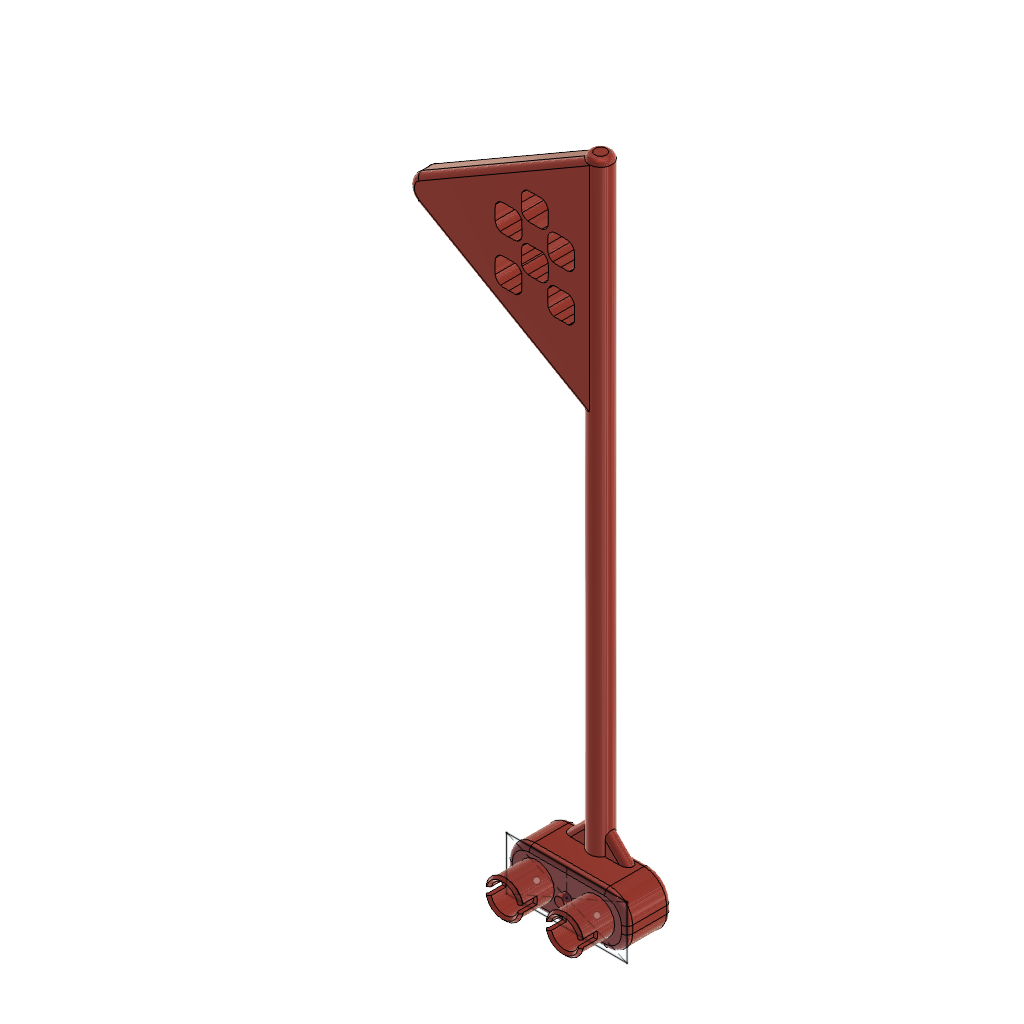
roversa_flag (Autodesk Fusion 360 design; units mm, degrees)
part number: 2026-09-13-09-05-21-145
Autodesk Fusion 360 part; units mm, degrees
sketch "Sketch1" plane through (0, 0, 0) normal (0, 1, 0) x (1, 0, 0)
  line L0 (8, -3.5) -> (-8, -3.5)
  line L1 (-8, -3.5) -> (-8, 3.5)
  line L2 (-8, 3.5) -> (8, 3.5)
  line L3 (8, 3.5) -> (8, -3.5)
  line L4 (8, -3.5) -> (-8, 3.5) construction
  line L5 (-8, -3.5) -> (8, 3.5) construction
  line L6 (0, -3.5) -> (0, 3.5) construction
  point P0 (-4, 0)
  point P1 (4, 0)
  dimension "d9" = 16
  dimension "d10" = 7
  dimension "d11" = 8
  constraint horizontal L0
  constraint perpendicular L0 L1
  constraint parallel L0 L2
  constraint parallel L1 L3
  constraint coincident L4 origin
  constraint coincident L5 origin
  constraint midpoint L0 L6.start
  constraint midpoint L2 L6.end
  constraint symmetric P0 P1 L6
  measures "d9" distance of L1.end L2.end
  measures "d10" distance of L0.end L1.end
  measures "d11" distance of P0 P1
extrude "Extrude1" add sketch "Sketch1" along normal blind 6
sketch "Sketch2" plane through (0, 0, 0) normal (0, 1, 0) x (1, 0, 0)
  circle A0 centre (-4, 0) radius 2.35
  circle A1 centre (-4, 0) radius 1.85
  dimension "d15" = 4.7
  dimension "d16" = 3.7
  constraint concentric A0 A1
  measures "d15" diameter of A0
  measures "d16" diameter of A1
extrude "Extrude2" add sketch "Sketch2" against normal blind 4.25
sketch "Sketch3" plane through (0, 0, 0) normal (0, 1, 0) x (1, 0, 0)
  circle A0 centre (4, 0) radius 2.35
  circle A1 centre (4, 0) radius 1.85
  dimension "d20" = 4.7
  dimension "d21" = 3.7
  constraint concentric A0 A1
  measures "d20" diameter of A0
  measures "d21" diameter of A1
extrude "Extrude3" add sketch "Sketch3" against normal blind 4.25
sketch "Sketch4" plane through (0, -4.25, 0) normal (0, -1, 0) x (1, 0, 0)
  circle A0 centre (-4, 0) radius 1.85
  circle A1 centre (-4, 0) radius 2.35
  circle A2 centre (-4, 0) radius 2.5
  dimension "d25" = 0.15
extrude "Extrude4" add sketch "Sketch4" along normal blind 1 draft -45 contours A1 | A2
sketch "Sketch5" plane through (0, -4.25, 0) normal (0, -1, 0) x (1, 0, 0)
  circle A0 centre (4, 0) radius 1.85
  circle A1 centre (4, 0) radius 2.35
  circle A2 centre (4, 0) radius 2.5
  dimension "d28" = 0.15
extrude "Extrude5" add sketch "Sketch5" along normal blind 1 draft -45 contours A1 | A2
ref_plane "WorkPlane1" through (-4, -4.575, 2.175) normal (0, 1, 0) x (-1, 0, 0)
sketch "Sketch6" plane through (0, -4.575, 0) normal (0, 1, 0) x (1, 0, 0)
  line L0 (-7.4125, -0.5) -> (-0.3625, -0.5)
  line L1 (-0.3625, -0.5) -> (-0.3625, 0.5)
  line L2 (-0.3625, 0.5) -> (-7.4125, 0.5)
  line L3 (-7.4125, 0.5) -> (-7.4125, -0.5)
  line L4 (-7.4125, -0.5) -> (-0.3625, 0.5) construction
  line L5 (-0.3625, -0.5) -> (-7.4125, 0.5) construction
  point P0 (-3.8875, 0)
  dimension "d32" = 1
  dimension "d33" = 7.05
  constraint horizontal L0
  constraint perpendicular L0 L1
  constraint parallel L0 L2
  constraint parallel L1 L3
  constraint coincident L4 P0
  constraint coincident L5 P0
  measures "d32" distance of L0.end L1.end
  measures "d33" distance of L0.start L0.end
extrude "Extrude6" cut sketch "Sketch6" along normal blind 2.3
sketch "Sketch7" plane through (0, -4.575, 0) normal (0, 1, 0) x (1, 0, 0)
  line L0 (0.5875, -0.5) -> (7.6375, -0.5)
  line L1 (7.6375, -0.5) -> (7.6375, 0.5)
  line L2 (7.6375, 0.5) -> (0.5875, 0.5)
  line L3 (0.5875, 0.5) -> (0.5875, -0.5)
  line L4 (0.5875, -0.5) -> (7.6375, 0.5) construction
  line L5 (7.6375, -0.5) -> (0.5875, 0.5) construction
  point P0 (4.1125, 0)
  dimension "d36" = 7.05
  dimension "d37" = 1
  constraint horizontal L0
  constraint perpendicular L0 L1
  constraint parallel L0 L2
  constraint parallel L1 L3
  constraint coincident L4 P0
  constraint coincident L5 P0
  measures "d36" distance of L0.start L0.end
  measures "d37" distance of L0.start L2.end
extrude "Extrude7" cut sketch "Sketch7" along normal blind 2.3
fillet "Fillet1" radius 3 4 edges at (8, 3, 3.5) (-8, 3, 3.5) (-8, 3, -3.5) (8, 3, -3.5)
sketch "Sketch8" plane through (0, 0, 3.5) normal (0, 0, 1) x (-1, 0, 0)
  line L0 (5, -6) -> (5, 0)
  line L1 (5, 0) -> (-5, 0)
  line L2 (-5, 0) -> (-5, -6)
  line L3 (-5, -6) -> (5, -6)
  circle A0 centre (0, -4.5) radius 1.5
  dimension "d45" = 3
  constraint tangent L3 A0
  measures "d45" diameter of A0
extrude "Extrude8" add sketch "Sketch8" along normal blind 80 contours A0
sketch "Sketch9" plane through (0, 6, 0) normal (0, 1, 0) x (-1, 0, 0)
  arc A0 (-8, -0.5) -> (-5, -3.5) centre (-5, -0.5) ccw
  line L0 (-5, -3.5) -> (5, -3.5)
  arc A1 (5, -3.5) -> (8, -0.5) centre (5, -0.5) ccw
  line L1 (8, -0.5) -> (8, 0.5)
  arc A2 (8, 0.5) -> (5, 3.5) centre (5, 0.5) ccw
  line L2 (5, 3.5) -> (0, 3.5)
  line L3 (0, 3.5) -> (-5, 3.5)
  arc A3 (-5, 3.5) -> (-8, 0.5) centre (-5, 0.5) ccw
  line L4 (-8, 0.5) -> (-8, -0.5)
  line L5 (0, 83.5) -> (25.9808, 68.5)
  line L6 (0, 83.5) -> (8.2765, 83.5) construction
  line L7 (25.9808, 68.5) -> (0, 53.5)
  line L8 (25.9808, 68.5) -> (15.4835, 68.5) construction
  line L9 (0, 53.5) -> (0, 83.5)
  line L10 (1.5, 83.5) -> (-1.5, 83.5)
  line L11 (-1.5, 3.5) -> (-1.5, 83.5)
  line L12 (-5, 3.5) -> (-1.5, 3.5)
  arc A4 (-5, 3.5) -> (-8, 0.5) centre (-5, 0.5) ccw
  line L13 (-8, -0.5) -> (-8, 0.5)
  arc A5 (-8, -0.5) -> (-5, -3.5) centre (-5, -0.5) ccw
  line L14 (5, -3.5) -> (-5, -3.5)
  arc A6 (5, -3.5) -> (8, -0.5) centre (5, -0.5) ccw
  line L15 (8, 0.5) -> (8, -0.5)
  arc A7 (8, 0.5) -> (5, 3.5) centre (5, 0.5) ccw
  line L16 (1.5, 3.5) -> (5, 3.5)
  line L17 (1.5, 3.5) -> (1.5, 83.5)
  point P0 (0, 83.5)
  dimension "d50" = 30
  dimension "d51" = 150
  dimension "d55" = 30
  constraint horizontal L6
  constraint horizontal L8
  constraint perpendicular L6 L9
  constraint midpoint L10 P0
  constraint coincident P0 L5.start
  measures "d50" angle of L5 L6
  measures "d51" angle of L7 L8
  measures "d55" distance of P0 L7.end
extrude "Extrude9" add sketch "Sketch9" against normal blind 3 contours L5 L7 L9 L17 | L5 L7 L17
fillet "Fillet3" radius 0.75 17 edges at (7.1213, 6, 2.6213) (8, 6, 0) (7.1213, 6, -2.6213) (0, 6, -3.5) (-7.1213, 6, -2.6213) (-8, 6, 0) (-7.1213, 6, 2.6213) (-2.5, 6, 3.5) (2.5, 6, 3.5) (-7.1213, 0, 2.6213) (-8, 0, 0) (-7.1213, 0, -2.6213) (0, 0, -3.5) (7.1213, 0, -2.6213) (8, 0, 0) (7.1213, 0, 2.6213) (0, 0, 3.5)
chamfer "Chamfer1" distance 0.15 angle 45 1 edges at (-4, -4.25, 2.35)
chamfer "Chamfer2" distance 0.15 angle 45 1 edges at (-4, -4.25, -2.35)
chamfer "Chamfer3" distance 0.15 angle 45 1 edges at (4, -4.25, -2.35)
chamfer "Chamfer4" distance 0.15 angle 45 1 edges at (4, -4.25, 2.35)
sketch "Sketch10" plane through (0, 0, 0) normal (0, 1, 0) x (1, 0, 0)
  circle A0 centre (0, 0) radius 0.65
  dimension "d66" = 1.3
  constraint coincident A0.centre origin
  measures "d66" diameter of A0
extrude "Extrude10" add sketch "Sketch10" against normal blind 1
ref_plane "WorkPlane2" through (0, 5.25, 0.375) normal (0, 1, 0) x (0, 0, 1)
sketch "Sketch11" plane through (0, 5.25, 0) normal (0, 1, 0) x (1, 0, 0)
  line L0 (-4.3507, -3.4546) -> (-1.3507, -3.4546)
  line L1 (-1.3507, -3.4546) -> (-1.3507, -6.4546)
  line L2 (-1.3507, -6.4546) -> (-4.3507, -3.4546)
  line L3 (-5, -3.5) -> (4.5424, -3.229) construction
  line L4 (4.5424, -3.229) -> (5, -3.5) construction
  line L5 (0, -3.5) -> (0, -6.024) construction
  line L6 (1.3507, -3.4546) -> (1.3507, -6.4546)
  line L7 (1.3507, -6.4546) -> (4.3507, -3.4546)
  line L8 (4.3507, -3.4546) -> (1.3507, -3.4546)
  dimension "d71" = 45
  dimension "d72" = 3
  constraint horizontal L0
  constraint perpendicular L0 L1
  constraint vertical L5
  constraint symmetric L0.start L5 L7.end
  constraint symmetric L0.end L5 L6.start
  constraint symmetric L1.end L5 L6.end
  measures "d71" angle of L1 L2
  measures "d72" distance of L0.start L0.end
extrude "Extrude11" add sketch "Sketch11" against normal blind 1.5
fillet "Fillet4" radius 0.75 4 edges at (2.8281, 5.25, 4.9773) (-2.8281, 5.25, 4.9773) (-2.8281, 3.75, 4.9773) (2.8281, 3.75, 4.9773)
fillet "Fillet5" radius 0.75 4 edges at (-12.9904, 6, 61) (-12.9904, 3, 61) (-12.9904, 6, 76) (-12.9904, 3, 76)
fillet "Fillet6" radius 0.75 1 edges at (1.3985, 5.0424, 83.5)
fillet "Fillet7" radius 2 3 edges at (-25.5414, 5.7803, 68.5) (-25.9808, 4.5, 68.5) (-25.5414, 3.2197, 68.5)
sketch "roversa-icon" plane through (0, 3, 0) normal (0, -1, 0) x (0, 0, -1)
  line L0 (-77.6583, 1.3985) -> (-77.6583, -15.6015)
  line L1 (-60.6583, -15.6015) -> (-60.6583, 1.3985)
  line L2 (-77.6583, -15.6015) -> (-60.6583, -15.6015)
  line L3 (-60.6583, 1.3985) -> (-77.6583, 1.3985)
  spline S0 degree 3 poles (-63.0001, -11.796) (-63.1468, -12.1963) (-63.447, -12.4351) (-63.89, -12.5038) knots 0 0 0 0 1 1 1 1
  spline S1 degree 3 poles (-63.89, -12.5038) (-64.2458, -12.559) (-65.6097, -12.527) (-65.7914, -12.4591) knots 0 0 0 0 1 1 1 1
  spline S2 degree 3 poles (-65.7914, -12.4591) (-66.1335, -12.3314) (-66.4173, -12.0056) (-66.4895, -11.6575) knots 0 0 0 0 1 1 1 1
  spline S3 degree 3 poles (-66.4895, -11.6575) (-66.5121, -11.5487) (-66.5212, -11.176) (-66.5147, -10.6238) knots 0 0 0 0 1 1 1 1
  spline S4 degree 3 poles (-66.5147, -10.6238) (-66.505, -9.8046) (-66.5008, -9.7523) (-66.4326, -9.6044) knots 0 0 0 0 1 1 1 1
  spline S5 degree 3 poles (-66.4326, -9.6044) (-66.3229, -9.3666) (-66.1659, -9.1969) (-65.9446, -9.0769) knots 0 0 0 0 1 1 1 1
  line L4 (-65.9446, -9.0769) -> (-65.7439, -8.9681)
  line L5 (-65.7439, -8.9681) -> (-64.7298, -8.9681)
  spline S6 degree 3 poles (-64.7298, -8.9681) (-63.7415, -8.9681) (-63.712, -8.9699) (-63.5707, -9.0395) knots 0 0 0 0 1 1 1 1
  spline S7 degree 3 poles (-63.5707, -9.0395) (-63.3477, -9.1494) (-63.1831, -9.3081) (-63.0638, -9.5282) knots 0 0 0 0 1 1 1 1
  line L6 (-63.0638, -9.5282) -> (-62.9551, -9.7287)
  line L7 (-62.9551, -9.7287) -> (-62.9472, -10.6794)
  spline S8 degree 3 poles (-62.9472, -10.6794) (-62.94, -11.5494) (-62.9445, -11.6442) (-63.0001, -11.796) knots 0 0 0 0 1 1 1 1
  spline S9 degree 3 poles (-62.9681, -4.7234) (-63.04, -5.013) (-63.2796, -5.2988) (-63.5707, -5.4423) knots 0 0 0 0 1 1 1 1
  spline S10 degree 3 poles (-63.5707, -5.4423) (-63.712, -5.5119) (-63.7415, -5.5137) (-64.7298, -5.5137) knots 0 0 0 0 1 1 1 1
  line L8 (-64.7298, -5.5137) -> (-65.7439, -5.5137)
  line L9 (-65.7439, -5.5137) -> (-65.9114, -5.4255)
  spline S11 degree 3 poles (-65.9114, -5.4255) (-66.1348, -5.3078) (-66.3183, -5.1185) (-66.4206, -4.9004) knots 0 0 0 0 1 1 1 1
  line L10 (-66.4206, -4.9004) -> (-66.5045, -4.7214)
  line L11 (-66.5045, -4.7214) -> (-66.5045, -3.7542)
  line L12 (-66.5045, -3.7542) -> (-66.5045, -2.7869)
  line L13 (-66.5045, -2.7869) -> (-66.4003, -2.5753)
  spline S12 degree 3 poles (-66.4003, -2.5753) (-66.2758, -2.3225) (-66.0808, -2.1389) (-65.8278, -2.0366) knots 0 0 0 0 1 1 1 1
  spline S13 degree 3 poles (-65.8278, -2.0366) (-65.6555, -1.967) (-65.6141, -1.9643) (-64.7139, -1.9643) knots 0 0 0 0 1 1 1 1
  line L14 (-64.7139, -1.9643) -> (-63.779, -1.9643)
  line L15 (-63.779, -1.9643) -> (-63.5992, -2.0486)
  spline S14 degree 3 poles (-63.5992, -2.0486) (-63.3587, -2.1613) (-63.1499, -2.3599) (-63.0429, -2.5777) knots 0 0 0 0 1 1 1 1
  line L16 (-63.0429, -2.5777) -> (-62.9551, -2.7566)
  line L17 (-62.9551, -2.7566) -> (-62.9495, -3.6915)
  spline S15 degree 3 poles (-62.9495, -3.6915) (-62.9465, -4.2057) (-62.9548, -4.67) (-62.9681, -4.7234) knots 0 0 0 0 1 1 1 1
  spline S16 degree 3 poles (-66.0446, -8.147) (-66.1116, -8.4683) (-66.3324, -8.7578) (-66.6313, -8.9159) knots 0 0 0 0 1 1 1 1
  line L18 (-66.6313, -8.9159) -> (-66.7897, -8.9998)
  line L19 (-66.7897, -8.9998) -> (-67.7586, -9.0093)
  spline S17 degree 3 poles (-67.7586, -9.0093) (-68.679, -9.0184) (-68.7364, -9.0156) (-68.9059, -8.9522) knots 0 0 0 0 1 1 1 1
  spline S18 degree 3 poles (-68.9059, -8.9522) (-69.1279, -8.8691) (-69.3617, -8.6624) (-69.4847, -8.4404) knots 0 0 0 0 1 1 1 1
  line L20 (-69.4847, -8.4404) -> (-69.5786, -8.2709)
  line L21 (-69.5786, -8.2709) -> (-69.5786, -7.2409)
  line L22 (-69.5786, -7.2409) -> (-69.5786, -6.2109)
  line L23 (-69.5786, -6.2109) -> (-69.4857, -6.0433)
  spline S19 degree 3 poles (-69.4857, -6.0433) (-69.3794, -5.8515) (-69.1831, -5.6586) (-68.998, -5.5642) knots 0 0 0 0 1 1 1 1
  spline S20 degree 3 poles (-68.998, -5.5642) (-68.7852, -5.4556) (-68.4723, -5.4271) (-67.6485, -5.4412) knots 0 0 0 0 1 1 1 1
  spline S21 degree 3 poles (-67.6485, -5.4412) (-66.9969, -5.4524) (-66.8639, -5.463) (-66.7422, -5.5131) knots 0 0 0 0 1 1 1 1
  spline S22 degree 3 poles (-66.7422, -5.5131) (-66.4321, -5.641) (-66.2217, -5.8512) (-66.0911, -6.1634) knots 0 0 0 0 1 1 1 1
  spline S23 degree 3 poles (-66.0911, -6.1634) (-66.0384, -6.2894) (-66.0307, -6.4054) (-66.0245, -7.1617) knots 0 0 0 0 1 1 1 1
  spline S24 degree 3 poles (-66.0245, -7.1617) (-66.0207, -7.6323) (-66.0298, -8.0757) (-66.0446, -8.147) knots 0 0 0 0 1 1 1 1
  spline S25 degree 3 poles (-69.1659, -11.8494) (-69.3105, -12.2009) (-69.6285, -12.4403) (-70.0349, -12.5033) knots 0 0 0 0 1 1 1 1
  spline S26 degree 3 poles (-70.0349, -12.5033) (-70.3916, -12.5587) (-71.758, -12.5279) (-71.9332, -12.4606) knots 0 0 0 0 1 1 1 1
  spline S27 degree 3 poles (-71.9332, -12.4606) (-72.23, -12.3466) (-72.4814, -12.0953) (-72.5959, -11.7981) knots 0 0 0 0 1 1 1 1
  spline S28 degree 3 poles (-72.5959, -11.7981) (-72.6384, -11.6878) (-72.6509, -11.5076) (-72.6611, -10.8517) knots 0 0 0 0 1 1 1 1
  spline S29 degree 3 poles (-72.6611, -10.8517) (-72.6745, -9.9997) (-72.6536, -9.7698) (-72.5421, -9.5393) knots 0 0 0 0 1 1 1 1
  spline S30 degree 3 poles (-72.5421, -9.5393) (-72.4582, -9.366) (-72.2454, -9.1551) (-72.0505, -9.0519) knots 0 0 0 0 1 1 1 1
  line L24 (-72.0505, -9.0519) -> (-71.892, -8.9681)
  line L25 (-71.892, -8.9681) -> (-70.9231, -8.9585)
  spline S31 degree 3 poles (-70.9231, -8.9585) (-69.9882, -8.9492) (-69.9477, -8.9514) (-69.7666, -9.0191) knots 0 0 0 0 1 1 1 1
  spline S32 degree 3 poles (-69.7666, -9.0191) (-69.5118, -9.1144) (-69.2503, -9.3748) (-69.1559, -9.6271) knots 0 0 0 0 1 1 1 1
  spline S33 degree 3 poles (-69.1559, -9.6271) (-69.0913, -9.7997) (-69.0874, -9.8636) (-69.0881, -10.736) knots 0 0 0 0 1 1 1 1
  spline S34 degree 3 poles (-69.0881, -10.736) (-69.0888, -11.6434) (-69.0904, -11.6656) (-69.1659, -11.8494) knots 0 0 0 0 1 1 1 1
  spline S35 degree 3 poles (-69.1571, -4.8629) (-69.2378, -5.0731) (-69.4788, -5.325) (-69.7053, -5.4361) knots 0 0 0 0 1 1 1 1
  spline S36 degree 3 poles (-69.7053, -5.4361) (-69.8612, -5.5125) (-69.8791, -5.5139) (-70.8168, -5.5233) knots 0 0 0 0 1 1 1 1
  spline S37 degree 3 poles (-70.8168, -5.5233) (-71.9246, -5.5345) (-71.995, -5.5213) (-72.2965, -5.2457) knots 0 0 0 0 1 1 1 1
  spline S38 degree 3 poles (-72.2965, -5.2457) (-72.6342, -4.9371) (-72.6786, -4.7404) (-72.6611, -3.6301) knots 0 0 0 0 1 1 1 1
  spline S39 degree 3 poles (-72.6611, -3.6301) (-72.6471, -2.7323) (-72.6357, -2.6713) (-72.4305, -2.3917) knots 0 0 0 0 1 1 1 1
  spline S40 degree 3 poles (-72.4305, -2.3917) (-72.3115, -2.2296) (-72.0993, -2.0782) (-71.892, -2.0075) knots 0 0 0 0 1 1 1 1
  spline S41 degree 3 poles (-71.892, -2.0075) (-71.7964, -1.9749) (-71.5394, -1.9643) (-70.8455, -1.9643) knots 0 0 0 0 1 1 1 1
  line L26 (-70.8455, -1.9643) -> (-69.9258, -1.9643)
  line L27 (-69.9258, -1.9643) -> (-69.7171, -2.067)
  spline S42 degree 3 poles (-69.7171, -2.067) (-69.4534, -2.1969) (-69.2458, -2.4147) (-69.1554, -2.6564) knots 0 0 0 0 1 1 1 1
  spline S43 degree 3 poles (-69.1554, -2.6564) (-69.0913, -2.8275) (-69.0874, -2.8925) (-69.089, -3.764) knots 0 0 0 0 1 1 1 1
  spline S44 degree 3 poles (-69.089, -3.764) (-69.0905, -4.6258) (-69.0952, -4.7017) (-69.1571, -4.8629) knots 0 0 0 0 1 1 1 1
  spline S45 degree 3 poles (-72.191, -8.1758) (-72.2687, -8.4954) (-72.4948, -8.7817) (-72.7802, -8.9222) knots 0 0 0 0 1 1 1 1
  spline S46 degree 3 poles (-72.7802, -8.9222) (-72.9356, -8.9986) (-72.9518, -8.9999) (-73.9077, -9.009) knots 0 0 0 0 1 1 1 1
  spline S47 degree 3 poles (-73.9077, -9.009) (-74.832, -9.0177) (-74.8861, -9.015) (-75.058, -8.9507) knots 0 0 0 0 1 1 1 1
  spline S48 degree 3 poles (-75.058, -8.9507) (-75.2779, -8.8684) (-75.538, -8.6251) (-75.6492, -8.3976) knots 0 0 0 0 1 1 1 1
  spline S49 degree 3 poles (-75.6492, -8.3976) (-75.7264, -8.2398) (-75.7267, -8.2353) (-75.7267, -7.2409) knots 0 0 0 0 1 1 1 1
  spline S50 degree 3 poles (-75.7267, -7.2409) (-75.7267, -6.2457) (-75.7264, -6.2421) (-75.649, -6.0842) knots 0 0 0 0 1 1 1 1
  spline S51 degree 3 poles (-75.649, -6.0842) (-75.5358, -5.8531) (-75.2871, -5.6178) (-75.0602, -5.5269) knots 0 0 0 0 1 1 1 1
  spline S52 degree 3 poles (-75.0602, -5.5269) (-74.8763, -5.4533) (-74.8459, -5.4511) (-73.9678, -5.4507) knots 0 0 0 0 1 1 1 1
  spline S53 degree 3 poles (-73.9678, -5.4507) (-73.1875, -5.4504) (-73.043, -5.4579) (-72.9061, -5.5059) knots 0 0 0 0 1 1 1 1
  spline S54 degree 3 poles (-72.9061, -5.5059) (-72.5605, -5.6271) (-72.2688, -5.9508) (-72.195, -6.295) knots 0 0 0 0 1 1 1 1
  spline S55 degree 3 poles (-72.195, -6.295) (-72.1575, -6.47) (-72.1542, -8.0243) (-72.191, -8.1758) knots 0 0 0 0 1 1 1 1
extrude "Extrude12" cut sketch "roversa-icon" against normal up to surface (3 mm away) contours S0 S1 S2 S3 S4 S5 L4 L5 S6 S7 L6 L7 S8 | S9 S10 L8 L9 S11 L10 L11 L12 L13 S12 S13 L14 L15 S14 L16 L17 S15 | S16 L18 L19 S17 S18 L20 L21 L22 L23 S19 S20 S21 S22 S23 S24 | S25 S26 S27 S28 S29 S30 L24 L25 S31 S32 S33 S34 | S35 S36 S37 S38 S39 S40 S41 L26 L27 S42 S43 S44 | S45 S46 S47 S48 S49 S50 S51 S52 S53 S54 S55
equation "pin_spacing = 8 mm"
equation "pin_diameter = 4.70 mm"
equation "retention_lip_diameter = 4.85 mm"
equation "pin_engagement_length = pin_length + separator_width"
equation "pin_relief_slot_width = 1 mm"
equation "pin_relief_slot_depth = 2.3 mm"
equation "flag_base_length = pin_spacing * 2"
equation "flag_base_width = 7 mm"
equation "d9 = flag_base_length"
equation "d10 = flag_base_width"
equation "d11 = pin_spacing"
equation "base_plate_thickness = 6 mm"
equation "d13 = base_plate_thickness"
equation "d15 = pin_diameter"
equation "d16 = pin_diameter - pin_wall_thickness"
equation "pin_wall_thickness = 1 mm"
equation "d18 = -pin_engagement_length"
equation "d20 = pin_diameter"
equation "d21 = pin_diameter - pin_wall_thickness"
equation "d22 = -pin_engagement_length"
equation "retention_lip_length = 1 mm"
equation "d25 = retention_lip_diameter - pin_diameter"
equation "d26 = retention_lip_length"
equation "d28 = retention_lip_diameter - pin_diameter"
equation "d29 = retention_lip_length"
equation "d32 = pin_relief_slot_width"
equation "d33 = pin_diameter * 1.5"
equation "d34 = pin_relief_slot_depth"
equation "d36 = pin_diameter * 1.5"
equation "d37 = pin_relief_slot_width"
equation "d38 = pin_relief_slot_depth"
equation "flag_base_corner_fillet = 3 mm"
equation "flag_height = 30 mm"
equation "d43 = flag_base_corner_fillet"
equation "global_fillet = 0.75 mm"
equation "d45 = flagpole_diameter"
equation "flagpole_diameter = 3 mm"
equation "flagpole_height = 80 mm"
equation "d48 = flagpole_height"
equation "d50 = flag_angle"
equation "d51 = 180 deg - flag_angle"
equation "d52 = -flagpole_diameter"
equation "flag_angle = 30 deg"
equation "d55 = flag_height"
equation "d59 = global_fillet"
equation "separator_width = 1 mm"
equation "pin_length = 3.25 mm"
equation "d66 = pin_spacing - pin_diameter - 2 mm"
equation "d67 = -separator_width"
equation "d69 = -global_fillet"
equation "d72 = flagpole_diameter"
equation "d73 = -flagpole_diameter / 2"
equation "d76 = global_fillet"
equation "d78 = global_fillet"
equation "big_fillet = 2 mm"
equation "d81 = global_fillet"
equation "d83 = big_fillet"
named bodies: "base-with-flag"
